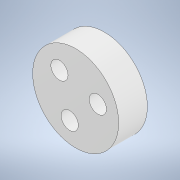
# Autodesk Inventor part: カム
Saved by Autodesk Inventor 2020.2 (Build 242310000, 310)
## iProperties
Created: 2020-03-20
Part Number: カム
Material: アセタール樹脂、白
Document SubType Name: Modeling
Designer: aoyam
Density: 1.425 g/cm^3
Appearance: 滑らか - 白
Author: aoyam
Autodesk Inventor part; units mm, degrees
ref_plane "YZ Plane" through (0, 0, 0) normal (1, 0, 0) x (0, 1, 0)
ref_plane "XZ Plane" through (0, 0, 0) normal (0, 1, 0) x (-1, 0, 0)
ref_plane "XY Plane" through (0, 0, 0) normal (0, 0, 1) x (1, 0, 0)
sketch "スケッチ1" plane through (0, 0, 0) normal (0, 0, 1) x (1, 0, 0)
  circle A0 centre (0, 0) radius 7.5
  circle A1 centre (-2.8284, 2.8284) radius 1.5
  circle A2 centre (-1.0353, -3.8637) radius 1.5
  circle A3 centre (3.8637, 1.0353) radius 1.5
  dimension "d0" = 15
  dimension "d1" = 3
  dimension "d2" = 4
  dimension "d5" = 360
  constraints: 4 centre point, 1 coincident, 7 other
  measures "d0" diameter of A0
  measures "d1" diameter of A1
  measures "d2" distance of A1.centre point (0, 0)
extrude "押し出し1" add sketch "スケッチ1" along normal blind 5
